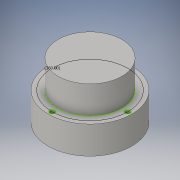
# Autodesk Inventor part: 7.2 part 2
Saved by Autodesk Inventor 2016 (Build 200138000, 138)
## iProperties
Created: 2017-03-14
Part Number: 7.2 part 2
Material: Generic
Document SubType Name: Modeling
Designer: 196918
Density: 1 g/cm^3
Appearance: Default
Author: 196918
Autodesk Inventor part; units mm, degrees
ref_plane "YZ Plane" through (0, 0, 0) normal (1, 0, 0) x (0, 1, 0)
ref_plane "XZ Plane" through (0, 0, 0) normal (0, 1, 0) x (-1, 0, 0)
ref_plane "XY Plane" through (0, 0, 0) normal (0, 0, 1) x (1, 0, 0)
sketch "Sketch1" plane through (0, 0, 0) normal (0, 1, 0) x (-1, 0, 0)
  circle A0 centre (0, 0) radius 19.05
  dimension "d0" = 38.1
  constraints: 1 centre point, 1 coincident
  measures "d0" diameter of A0
extrude "Extrusion1" add sketch "Sketch1" along normal blind 12.7
sketch "Sketch2" plane through (0, 12.7, 0) normal (0, 1, 0) x (1, 0, 0)
  circle A0 centre (-17.2164, 0) radius 1.2279
  circle A1 centre (0, -17.2164) radius 1.2279
  circle A2 centre (17.2164, 0) radius 1.2279
  circle A3 centre (0, 17.2164) radius 1.2279
  circle A4 centre (0, 0) radius 14.5525
  dimension "d5" = 360
  constraints: 5 centre point, 3 coincident, 11 other
extrude "Extrusion2" add sketch "Sketch2" along normal blind 12.7 contours A4
extrude "Extrusion3" cut sketch "Sketch2" against normal up to next contours A0 | A1 | A2 | A3
body "Solid1"
